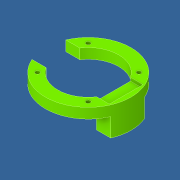
# Autodesk Inventor part: EncoderDistanz
Saved by Autodesk Inventor 2016 (Build 200138000, 138)
## iProperties
Created: 2015-10-04
Part Number: EncoderDistanz
Material: ABS-Kunststoff
Document SubType Name: Modeling
Designer: 4ndreas
Density: 1.06 g/cm^3
Appearance: Glatt - grün
Mass: 7.44836 g
Surface Area: 40.5446 cm^2
Volume: 7.02675 cm^3
Author: 4ndreas
Autodesk Inventor part; units mm, degrees
ref_plane "YZ Plane" through (0, 0, 0) normal (1, 0, 0) x (0, 1, 0)
ref_plane "XZ Plane" through (0, 0, 0) normal (0, 1, 0) x (-1, 0, 0)
ref_plane "XY Plane" through (0, 0, 0) normal (0, 0, 1) x (1, 0, 0)
sketch "Skizze1" plane through (0, 0, 0) normal (0, 0, 1) x (1, 0, 0)
  circle A0 centre (-15, -15) radius 1.25 projected
  circle A1 centre (15, -15) radius 1.25 projected
  line L0 (23.2671, -10) -> (14.9666, -10) projected
  arc A2 (-14.9666, -10) -> (14.9666, -10) centre (0, 0) ccw projected
  line L1 (-14.9666, -10) -> (-23.2671, -10) projected
  arc A3 (-23.2671, -10) -> (23.2671, -10) centre (0, 0) ccw projected
  circle A4 centre (-15, 15) radius 1.25 projected
  circle A5 centre (15, 15) radius 1.25 projected
  line L2 (14.9666, 10) -> (23.2671, 10) projected
  arc A6 (23.2671, 10) -> (-23.2671, 10) centre (0, 0) ccw projected
  line L3 (-23.2671, 10) -> (-14.9666, 10) projected
  arc A7 (14.9666, 10) -> (-14.9666, 10) centre (0, 0) ccw projected
  point P0 (0, 0)
extrude "Extrusion1" add sketch "Skizze1" along normal blind 6
sketch "Skizze2" plane through (14.9666, -10, 0) normal (0, 1, 0) x (1, 0, 0)
  line L0 (0, 6) -> (0, 0) projected
  line L1 (8.3004, 0) -> (0, 0) projected
  line L2 (8.3004, 8.2705) -> (8.3004, 0) projected
  arc A0 (8.3004, 8.2705) -> (10.8169, 11) centre (1.6243, 16.9504) ccw projected
  line L3 (10.8169, 11) -> (0, 11) projected
  line L4 (0, 6) -> (0, 11) projected
  line L5 (8.3004, 0) -> (0, 0) projected
  line L6 (0, 0) -> (0, -6) projected
  line L7 (8.3004, -6) -> (0, -6) projected
  line L8 (8.3004, 0) -> (8.3004, -6) projected
  point P0 (-14.9666, 0)
extrude "Extrusion2" add sketch "Skizze2" along normal up to surface (20 mm away)
sketch "Skizze3" plane through (0, 0, 6) normal (0, 0, 1) x (1, 0, 0)
  arc A0 (23.2671, -10) -> (23.2671, 10) centre (0, 0) ccw
  circle A1 centre (-15, 15) radius 1.25 projected
  circle A2 centre (15, 15) radius 1.25 projected
  circle A3 centre (15, -15) radius 1.25 projected
  circle A4 centre (-15, -15) radius 1.25 projected
  arc A5 (-14.9666, -10) -> (14.9666, -10) centre (0, 0) ccw projected
  line L0 (-14.9666, -10) -> (-23.2671, -10) projected
  arc A6 (-23.2671, -10) -> (23.2671, -10) centre (0, 0) ccw projected
  line L1 (23.2671, -10) -> (23.2671, 10) projected
  arc A7 (23.2671, 10) -> (-23.2671, 10) centre (0, 0) ccw projected
  line L2 (-23.2671, 10) -> (-14.9666, 10) projected
  arc A8 (14.9666, 10) -> (-14.9666, 10) centre (0, 0) ccw projected
  line L3 (14.9666, -10) -> (14.9666, 10) projected
  constraints: 2 point on circle, 1 centre point, 1 coincident
extrude "Extrusion3" add sketch "Skizze3" against normal up to surface (17 mm away) contours L1 A0
sketch "Skizze4" plane through (0, 0, 6) normal (0, 0, 1) x (1, 0, 0)
  circle A0 centre (-15, 15) radius 1.25 projected
  circle A1 centre (15, 15) radius 1.25 projected
  circle A2 centre (15, -15) radius 1.25 projected
  circle A3 centre (-15, -15) radius 1.25 projected
  arc A4 (-14.9666, -10) -> (14.9666, -10) centre (0, 0) ccw projected
  line L0 (-14.9666, -10) -> (-23.2671, -10) projected
  arc A5 (-23.2671, -10) -> (-23.2671, 10) centre (0, 0) ccw projected
  line L1 (-23.2671, 10) -> (-14.9666, 10) projected
  arc A6 (14.9666, 10) -> (-14.9666, 10) centre (0, 0) ccw projected
  line L2 (14.9666, -10) -> (14.9666, 10) projected
  line L3 (14.9666, 10) -> (22.4666, 10)
  line L4 (22.4666, 10) -> (22.4666, -10)
  line L5 (22.4666, -10) -> (14.9666, -10)
  line L6 (14.9666, -10) -> (14.9666, 10)
  point P0 (0, 0)
  dimension "d6" = 7.5
  constraints: 8 end point, 2 parallel, 1 horizontal, 1 perpendicular
  measures "d6" distance between parallel lines of L2 L4
extrude "Extrusion4" cut sketch "Skizze4" against normal blind 2 contours L2 L3 L4 L5
sketch "Skizze6" plane through (25.7835, -10, -11) normal (0, 0, -1) x (-1, 0, 0)
  circle A0 centre (25.7835, 10) radius 25.325
  arc A1 (2.5165, 0) -> (49.0506, 0) centre (25.7835, 10) ccw projected
  circle A2 centre (25.7835, 10) radius 35.325
  dimension "d9" = 10
  constraints: 2 centre point, 2 coincident, 1 concentric
  measures "d9" radial gap between concentric circles of A2 A0
extrude "Extrusion5" cut sketch "Skizze6" against normal through all
